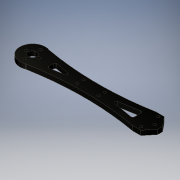
# Autodesk Inventor part: MotorLink
Saved by Autodesk Inventor 2018 (Build 220112000, 112)
## iProperties
Created: 2019-01-19
Part Number: MotorLink
Material: Generic
Document SubType Name: Modeling
Designer: anirudh
Density: 1 g/cm^3
Appearance: Gunmetal
Author: anirudh
Autodesk Inventor part; units mm, degrees
ref_plane "YZ Plane" through (0, 0, 0) normal (1, 0, 0) x (0, 1, 0)
ref_plane "XZ Plane" through (0, 0, 0) normal (0, 1, 0) x (-1, 0, 0)
ref_plane "XY Plane" through (0, 0, 0) normal (0, 0, 1) x (1, 0, 0)
sketch "Sketch1" plane through (0, 0, 0) normal (0, 1, 0) x (-1, 0, 0)
  arc A0 (127.4327, -29.2843) -> (127.4327, -1.1957) centre (133.35, -15.24) ccw
  circle A1 centre (133.35, -15.24) radius 5
  circle A2 centre (141.15, -15.24) radius 1.65
  circle A3 centre (133.35, -24.54) radius 1.65
  circle A4 centre (133.35, -5.94) radius 1.65
  circle A5 centre (125.55, -15.24) radius 1.65
  line L0 (7.62, -15.24) -> (7.62, -8.89)
  line L1 (7.62, -8.89) -> (7.62, -21.59)
  line L2 (44.6065, -15.24) -> (7.62, -8.89)
  line L3 (44.6065, -15.24) -> (7.62, -21.59)
  line L4 (111.2, -15.24) -> (111.2, -10.16)
  line L5 (111.2, -10.16) -> (111.2, -20.32)
  line L6 (111.2, -20.32) -> (82.7065, -15.24)
  line L7 (82.7065, -15.24) -> (111.2, -10.16)
  line L8 (-19, -18.24) -> (-10, -29.24)
  line L9 (-10, -29.24) -> (0, -29.24)
  line L10 (0, -1.24) -> (-10, -1.24)
  line L11 (0, -1.24) -> (-10, -1.24)
  line L12 (-10, -1.24) -> (-19, -12.24)
  line L13 (-10, -1.24) -> (-19, -12.24)
  line L14 (-19, -12.24) -> (-19, -18.24)
  line L15 (-19, -12.24) -> (-19, -18.24)
  line L16 (-19, -18.24) -> (-10, -29.24)
  circle A6 centre (-6.5, -25.49) radius 1.65
  circle A7 centre (-6.5, -25.49) radius 1.65
  circle A8 centre (-6.5, -4.99) radius 1.65
  circle A9 centre (-6.5, -4.99) radius 1.65
  arc A10 (0, -1.24) -> (127.4327, -1.1957) centre (63.5946, 348.7462) ccw
  arc A11 (127.4327, -29.2843) -> (0, -29.24) centre (63.5946, -379.2262) ccw
  circle A12 centre (-12.65, -15.24) radius 1.65
  point P0 (0, 0)
  constraints: 34 end point, 13 centre point, 6 point on circle, 3 coincident, 2 collinear, 1 horizontal
extrude "Extrusion2" add sketch "Sketch1" along normal blind 5.588
fillet "Fillet2" radius 1.905 8 edges at (-127.4327, 2.794, -1.1957) (-7.62, 2.794, -21.59) (-7.62, 2.794, -8.89) (-44.6065, 2.794, -15.24) (-111.2, 2.794, -20.32) (-111.2, 2.794, -10.16) (-82.7065, 2.794, -15.24) (-127.4327, 2.794, -29.2843)
sketch "Sketch3" plane through (0, 5.588, 0) normal (0, 1, 0) x (1, 0, 0)
  circle A0 centre (-76.4433, 11.43) radius 1.5
  circle A1 centre (-76.4433, 19.05) radius 1.5
  circle A2 centre (-50.7893, 11.43) radius 1.5
  circle A3 centre (-50.7893, 19.05) radius 1.5
  point P0 (0, 0)
  dimension "d49" = 3
  dimension "d50" = 3
  dimension "d52" = 3
  constraints: 4 centre point
  measures "d49" diameter of A0
  measures "d50" diameter of A1
  measures "d52" diameter of A3
extrude "Extrusion3" cut sketch "Sketch3" against normal blind 5.588
body "Solid2"
